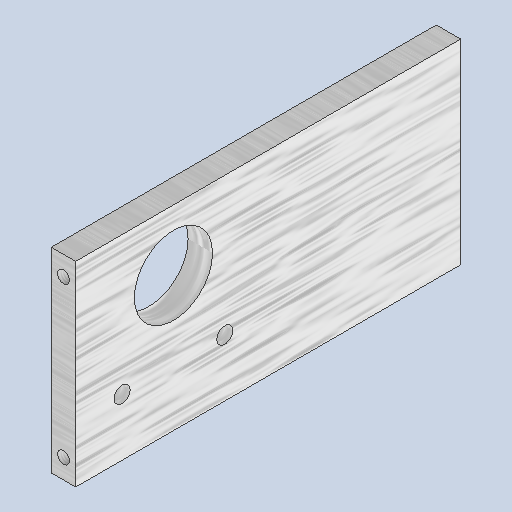
# Autodesk Inventor part: shoulder1_verticval_right_cover
Saved by Autodesk Inventor 2024 (Build 280153000, 153)
## iProperties
Created: 2025-08-06
Part Number: shoulder1_verticval_right_cover
Material: アルミニウム 5052
Document SubType Name: Modeling
Designer: HosodaLab2
Density: 2.68 g/cm^3
Appearance: サテン - ブラシ仕上げ 重厚
Author: HosodaLab2
Autodesk Inventor part; units mm, degrees
ref_plane "YZ Plane" through (0, 0, 0) normal (1, 0, 0) x (0, 1, 0)
ref_plane "XZ Plane" through (0, 0, 0) normal (0, 1, 0) x (-1, 0, 0)
ref_plane "XY Plane" through (0, 0, 0) normal (0, 0, 1) x (1, 0, 0)
sketch "スケッチ2" plane through (0, 0, 0) normal (0, 1, 0) x (-1, 0, 0)
  line L0 (0, 0) -> (-78.8, 0)
  line L1 (-78.8, 0) -> (-78.8, -40)
  line L2 (-78.8, -40) -> (0, -40)
  line L3 (0, -40) -> (0, 0)
  dimension "d0" = 78.8
  dimension "d1" = 40
  constraints: 8 end point, 2 parallel, 1 horizontal, 1 perpendicular
  measures "d0" distance of L2.end L1.end
  measures "d1" distance of L1.end L0.end
extrude "押し出し1" add sketch "スケッチ2" along normal blind 5
sketch "スケッチ4" plane through (0, 0, -40) normal (-1, 0, 0) x (0, 0, 1)
  line L0 (0, 0) -> (0, 5) construction
  line L1 (0, 2.5) -> (40, 2.5) construction
  line L2 (40, 0) -> (40, 5) construction
  point P0 (4, 2.5)
  point P1 (36, 2.5)
  dimension "d4" = 4
  dimension "d5" = 4
  constraints: 2 end point, 2 midpoint, 2 point on line
  measures "d4" distance from line of L2 point (36, 2.5)
  measures "d5" distance from line of point (4, 2.5) L0
hole "穴1" at (0, 2.5, -36) at (0, 2.5, -4) direction (1, 0, 0) diameter 2.459 depth 12 thread size "M3x0.5" class "6H" standard "ISO Metric profile"
sketch "スケッチ5" plane through (78.8, 0, 0) normal (1, 0, 0) x (0, 0, -1)
  line L0 (0, 0) -> (0, 5) construction
  line L1 (0, 2.5) -> (39.9198, 2.5) construction
  circle A0 centre (4, 2.5) radius 1.2295 construction
  circle A1 centre (36, 2.5) radius 1.2295 projected
  constraints: 2 coincident, 2 end point, 1 horizontal, 1 midpoint
hole "穴2" at (78.8, 2.5, -4) at (78.8, 2.5, -36) direction (-1, 0, 0) diameter 2.459 depth 12 thread size "M3x0.5" class "6H" standard "ISO Metric profile"
sketch "スケッチ6" plane through (0, 5, 0) normal (0, 1, 0) x (1, 0, 0)
  line L0 (78.8, 0) -> (78.8, 40) construction
  line L1 (0, 40) -> (0, 0) construction
  line L2 (0, 0) -> (78.8, 0) construction
  point P0 (58.8, 12.5)
  dimension "d20" = 20
  dimension "d21" = 12.5
  measures "d20" distance from line of L0 point (58.8, 12.5)
  measures "d21" distance from line of L2 point (58.8, 12.5)
hole "穴3" at (58.8, 5, -12.5) direction (0, -1, 0) diameter 16 end through all
sketch "スケッチ7" plane through (0, 5, 0) normal (0, 1, 0) x (1, 0, 0)
  line L0 (78.8, 0) -> (78.8, 40) construction
  line L1 (78.8, 28.3) -> (0, 28.3) construction
  line L2 (0, 40) -> (0, 0) construction
  circle A0 centre (58.8, 12.5) radius 8 construction
  point P0 (69.3, 28.3)
  point P1 (48.3, 28.3)
  dimension "d29" = 15.8
  dimension "d30" = 10.5
  dimension "d31" = 10.5
  constraints: 4 point on line, 2 end point, 1 horizontal
  measures "d29" distance from line of L1 A0.centre
  measures "d30" horizontal distance of point (69.3, 28.3) A0.centre
  measures "d31" horizontal distance of point (48.3, 28.3) A0.centre
hole "穴4" at (69.3, 5, -28.3) at (48.3, 5, -28.3) direction (0, -1, 0) diameter 3.3 end through all
